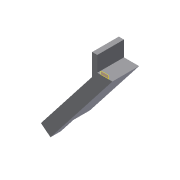
# Autodesk Inventor part: arm stop
Saved by Autodesk Inventor 2018 (Build 220112000, 112)
## iProperties
Created: 2018-12-28
Part Number: arm stop
Material: Generic
Document SubType Name: Modeling
Designer: ball
Density: 1 g/cm^3
Appearance: Default
Author: ball
Autodesk Inventor part; units mm, degrees
ref_plane "YZ Plane" through (0, 0, 0) normal (1, 0, 0) x (0, 1, 0)
ref_plane "XZ Plane" through (0, 0, 0) normal (0, 1, 0) x (-1, 0, 0)
ref_plane "XY Plane" through (0, 0, 0) normal (0, 0, 1) x (1, 0, 0)
ref_plane "Work Plane1" through (0, 0, 0) normal (0, 0, 1) x (1, 0, 0)
sketch "Sketch1" plane through (0, 0, 0) normal (0, 0, 1) x (1, 0, 0)
  line L0 (4.1292, -9.5377) -> (6.4068, -9.5377) construction
  line L1 (9.525, -8.413) -> (9.525, -7.4355) construction
  line L2 (-6.4068, 9.5123) -> (-4.1292, 9.5123) construction
  line L3 (-9.525, 4.1165) -> (-9.525, 6.3941) construction
  line L4 (9.3027, -9.3631) -> (-67.3225, -107.4389) construction
  line L5 (9.1663, -9.5377) -> (-67.3225, -107.4389)
  line L6 (-67.3225, -107.4389) -> (-79.1518, -98.1969)
  line L7 (4.9998, 9.5123) -> (-79.1518, -98.1969) construction
  line L8 (9.1663, -9.5377) -> (-9.5238, -9.5377)
  line L9 (-9.5238, -9.5377) -> (-9.5238, 9.5123)
  line L10 (-9.5238, 9.5123) -> (-15.8738, 9.5123)
  line L11 (-15.8738, 9.5123) -> (-15.8738, -17.2048)
  line L12 (-15.8738, -17.2048) -> (-79.1518, -98.1969)
  point P0 (0, 0)
  dimension "d0" = 124.46
  dimension "d1" = 52
  dimension "d5" = 6.35
  constraints: 26 end point, 4 point on line, 3 horizontal, 3 perpendicular, 2 collinear, 2 vertical, 1 parallel, 8 other
  measures "d0" distance of L4.start L4.end
  measures "d1" angle of L0 L4
  measures "d5" distance of L9.end L10.end
ref_plane "Work Plane2" through (-4.445, -9.144, -33.02) normal (0, 0, -1) x (0, 1, 0)
extrude "Extrusion1" add sketch "Sketch1" against normal up to surface (33.02 mm away)
sketch "Sketch2" plane through (-67.3225, -107.4389, -33.02) normal (-0.6156615, -0.7880108, 0) x (0.7880108, -0.6156615, 0)
  line L0 (0, 33.02) -> (0, 0) projected
  line L1 (-15.0116, 33.02) -> (-15.0116, 0) projected
  line L2 (0, 0) -> (-15.0116, 0)
  line L3 (-15.0116, 0) -> (-15.0116, 26.67)
  line L4 (-15.0116, 26.67) -> (0, 26.67)
  line L5 (0, 26.67) -> (0, 0)
  line L6 (-15.0116, 33.02) -> (0, 33.02) projected
  point P0 (-13.0951, 33.02)
  dimension "d19" = 6.35
  constraints: 8 end point, 2 parallel, 1 horizontal, 1 perpendicular, 1 point on line
  measures "d19" distance between parallel lines of L6 L4
extrude "Extrusion2" cut sketch "Sketch2" against normal blind 25.4 contours L0 L2 L1 L4
sketch "Sketch3" plane through (-67.3225, -107.4389, -6.35) normal (0, 0, -1) x (-0.7880108, 0.6156615, 0)
  line L0 (19.8882, 12.0904) -> (19.8882, 3.175) construction
  line L1 (0, 25.4) -> (15.0116, 25.4) construction
  line L2 (15.0116, 0) -> (0, 0) construction
  line L3 (0, 0) -> (19.8882, 0) construction
  line L4 (19.8882, 0) -> (19.8882, 25.4) construction
  line L5 (19.8882, 25.4) -> (0, 25.4) construction
  line L6 (0, 25.4) -> (0, 0) construction
  line L7 (15.0116, 0) -> (19.8882, 0)
  line L8 (19.8882, 0) -> (19.8882, 25.4)
  line L9 (19.8882, 25.4) -> (15.0116, 25.4)
  line L10 (15.0116, 25.4) -> (15.0116, 0)
  point P0 (13.0951, 126.1109)
  constraints: 18 end point, 4 parallel, 2 horizontal, 2 perpendicular, 1 vertical, 2 other
extrude "Extrusion3" add sketch "Sketch3" against normal up to surface (6.35 mm away)
sketch "Sketch4" plane through (0, 0, 0) normal (0, 0, 1) x (1, 0, 0)
  circle A0 centre (-72.9652, -90.7738) radius 1.1938 construction
  circle A1 centre (-65.4594, -96.6379) radius 1.1938 construction
  line L0 (-72.9652, -90.7738) -> (-65.3603, -81.0399) construction
  line L1 (-82.9946, -95.1945) -> (-67.3568, -75.1791) construction
  line L2 (-72.9652, -90.7738) -> (-77.2928, -96.3128) construction
  line L3 (-76.0928, -94.7769) -> (-69.8376, -86.7707) construction
  line L4 (-74.8518, -95.7464) -> (-68.5967, -87.7402)
  line L5 (-71.0786, -85.8011) -> (-77.3337, -93.8073)
  arc A2 (-77.3337, -93.8073) -> (-74.8518, -95.7464) centre (-76.0928, -94.7769) ccw
  arc A3 (-68.5967, -87.7402) -> (-71.0786, -85.8011) centre (-69.8376, -86.7707) ccw
  line L6 (-65.4594, -96.6379) -> (-58.3873, -87.5861) construction
  line L7 (-67.3225, -107.4389) -> (9.1663, -9.5377) construction
  line L8 (-65.4594, -96.6379) -> (-69.0558, -101.2411) construction
  line L9 (-68.587, -100.641) -> (-62.3318, -92.6349) construction
  line L10 (-67.346, -101.6106) -> (-61.0909, -93.6044)
  line L11 (-63.5728, -91.6653) -> (-69.8279, -99.6715)
  arc A4 (-69.8279, -99.6715) -> (-67.346, -101.6106) centre (-68.587, -100.641) ccw
  arc A5 (-61.0909, -93.6044) -> (-63.5728, -91.6653) centre (-62.3318, -92.6349) ccw
  point P0 (0, 0)
  dimension "d13" = 5.08
  dimension "d14" = 3.1496
  dimension "d15" = 5.08
  dimension "d16" = 3.1496
  constraints: 24 end point, 8 point on circle, 8 tangent, 6 centre point, 6 parallel, 2 midpoint, 2 point on line, 4 other
  measures "d13" distance of L0.start L3.end
  measures "d14" diameter of A3
  measures "d15" distance of L6.start L9.end
  measures "d16" diameter of A5
extrude "Extrusion4" cut sketch "Sketch4" against normal through all
sketch "Sketch5" plane through (-67.3225, -107.4389, -6.35) normal (0, 0, -1) x (-0.7880108, 0.6156615, 0)
  arc A0 (6.7564, 14.7384) -> (3.6068, 14.7384) centre (5.1816, 14.7384) ccw projected
  arc A1 (3.6068, 4.5784) -> (6.7564, 4.5784) centre (5.1816, 4.5784) ccw projected
  line L0 (5.1816, 14.7384) -> (5.1816, 4.5784) construction
  line L1 (1.6256, 14.7384) -> (1.6256, 4.5784)
  line L2 (8.7376, 4.5784) -> (8.7376, 14.7384)
  arc A2 (8.7376, 14.7384) -> (1.6256, 14.7384) centre (5.1816, 14.7384) ccw
  arc A3 (1.6256, 4.5784) -> (8.7376, 4.5784) centre (5.1816, 4.5784) ccw
  arc A4 (16.2814, 14.7384) -> (13.1318, 14.7384) centre (14.7066, 14.7384) ccw projected
  arc A5 (13.1318, 4.5784) -> (16.2814, 4.5784) centre (14.7066, 4.5784) ccw projected
  line L3 (14.7066, 14.7384) -> (14.7066, 4.5784) construction
  line L4 (11.1506, 14.7384) -> (11.1506, 4.5784)
  line L5 (18.2626, 4.5784) -> (18.2626, 14.7384)
  arc A6 (18.2626, 14.7384) -> (11.1506, 14.7384) centre (14.7066, 14.7384) ccw
  arc A7 (11.1506, 4.5784) -> (18.2626, 4.5784) centre (14.7066, 4.5784) ccw
  point P0 (13.0951, 126.1109)
  point P1 (5.1816, 9.6584)
  point P2 (14.7066, 9.6584)
  dimension "d20" = 7.112
  dimension "d21" = 7.112
  constraints: 16 end point, 8 point on circle, 8 tangent, 4 centre point, 3 parallel, 2 midpoint, 1 vertical
  measures "d20" diameter of A3
  measures "d21" diameter of A7
extrude "Extrusion5" cut sketch "Sketch5" against normal blind 3.556
sketch "Sketch6" plane through (-9.5238, -9.5377, 0) normal (0, 1, 0) x (1, 0, 0)
  arc A0 (9.5065, 4.7921) -> (10.7406, 4.301) centre (9.5238, 3.0396) ccw construction
  arc A1 (9.5065, 31.7329) -> (10.7406, 31.2417) centre (9.5238, 29.9804) ccw construction
  circle A2 centre (9.5238, 29.9804) radius 1.9685
  circle A3 centre (9.5238, 3.0396) radius 1.9685
  point P0 (9.5238, 0)
  dimension "d24" = 3.937
  dimension "d25" = 3.937
  constraints: 4 centre point, 4 point on circle, 2 coincident, 8 other
  measures "d24" diameter of A2
  measures "d25" diameter of A3
extrude "Extrusion6" cut sketch "Sketch6" against normal through all
sketch "Sketch7" plane through (9.1663, -9.5377, 0) normal (0.7880108, -0.6156615, 0) x (0, 0, -1)
  line L0 (33.02, -98.8385) -> (33.02, 0) construction
  line L1 (33.02, -9.525) -> (0, -9.525) construction
  point P0 (0, 1.8725)
  constraints: 2 end point, 1 perpendicular, 1 point on line
sketch "Sketch8" plane through (9.1663, -9.5377, -33.02) normal (0, 0, -1) x (-1, 0, 0)
  line L0 (11.1348, 0) -> (11.1348, -14.2519) construction
  line L1 (60.851, -77.8858) -> (0, 0) construction
  line L2 (11.1348, -7.62) -> (5.9534, -7.62) construction
  line L3 (0, 0) -> (18.6902, 0) construction
  line L4 (7.1978, 0) -> (7.1978, -9.2128) construction
  line L5 (14.4368, 0) -> (14.4368, -14.2519) construction
  line L6 (5.9534, -7.62) -> (14.4368, -7.62)
  line L7 (76.4888, -97.9012) -> (0, 0) projected
  line L8 (14.4368, -18.4783) -> (5.9534, -7.62)
  line L9 (14.4368, -18.4783) -> (14.4368, -7.62)
  point P0 (9.1663, 9.5377)
  dimension "d28" = 7.62
  dimension "d29" = 3.302
  constraints: 10 end point, 5 point on line, 1 collinear, 1 horizontal, 1 parallel
  measures "d28" distance between parallel lines of L3 L2
  measures "d29" distance between parallel lines of L0 L5
extrude "Extrusion7" cut sketch "Sketch8" against normal blind 8.763
sketch "Sketch9" plane through (0, 0, 0) normal (0, 0, 1) x (1, 0, 0)
  line L0 (3.2129, -17.1577) -> (-5.2705, -17.1577) construction
  line L1 (-5.2705, -17.1577) -> (-5.2705, -28.016) construction
  line L2 (3.2129, -17.1577) -> (-5.2705, -28.016)
  line L3 (-67.3225, -107.4389) -> (9.1663, -9.5377) projected
  line L4 (3.2129, -17.1577) -> (-5.2705, -17.1577) projected
  line L5 (-5.2705, -28.016) -> (-5.2705, -17.1577)
  point P0 (0, 0)
  constraints: 4 end point, 1 collinear, 1 vertical
extrude "Extrusion8" cut sketch "Sketch9" against normal blind 8.763
body "Solid1"
